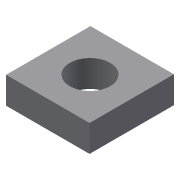
# Autodesk Inventor part: 00_Huawei_P20_Lens
Saved by Autodesk Inventor 2019 (Build 230136000, 136)
## iProperties
Created: 2019-08-19
Part Number: 00_Huawei_P20_Lens
Material: Generic
Document SubType Name: Modeling
Designer: diederichbenedict
Density: 1 g/cm^3
Appearance: Default
Author: diederichbenedict
Autodesk Inventor part; units mm, degrees
ref_plane "YZ Plane" through (0, 0, 0) normal (1, 0, 0) x (0, 1, 0)
ref_plane "XZ Plane" through (0, 0, 0) normal (0, 1, 0) x (-1, 0, 0)
ref_plane "XY Plane" through (0, 0, 0) normal (0, 0, 1) x (1, 0, 0)
sketch "Sketch1" plane through (0, 0, 0) normal (0, 1, 0) x (-1, 0, 0)
  line L0 (-4.675, 4.725) -> (4.675, 4.725)
  line L1 (4.675, 4.725) -> (4.675, -4.725)
  line L2 (4.675, -4.725) -> (-4.675, -4.725)
  line L3 (-4.675, -4.725) -> (-4.675, 4.725)
  line L4 (-4.675, 4.725) -> (4.675, -4.725) construction
  line L5 (4.675, 4.725) -> (-4.675, -4.725) construction
  circle A0 centre (0, 0) radius 2.2628
  dimension "d0" = 9.35
  dimension "d1" = 9.45
  constraints: 12 end point, 2 midpoint, 2 parallel, 1 centre point, 1 coincident, 1 horizontal, 1 perpendicular
  measures "d0" distance of L1.end L2.end
  measures "d1" distance of L0.end L1.end
extrude "Extrusion1" add sketch "Sketch1" along normal blind 3
sketch "Sketch2" plane through (0, 3, 0) normal (0, 1, 0) x (1, 0, 0)
  circle A0 centre (0, 0) radius 2.2628 projected
  line L0 (-4.675, -4.725) -> (4.675, -4.725) projected
  line L1 (4.675, -4.725) -> (4.675, 4.725) projected
  line L2 (4.675, 4.725) -> (-4.675, 4.725) projected
  line L3 (-4.675, 4.725) -> (-4.675, -4.725) projected
  circle A1 centre (0, 0) radius 2.5
  dimension "d4" = 5
  constraints: 1 centre point, 1 coincident
  measures "d4" diameter of A1
extrude "Extrusion2" add sketch "Sketch2" along normal blind 1.5 contours A0 | A1
body "Solid1"
